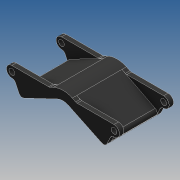
# Autodesk Inventor part: Front guard v2
Saved by Autodesk Inventor 2017 (Build 210142000, 142)
## iProperties
Created: 2017-07-08
Part Number: Front guard v2
Material: Generic
Document SubType Name: Modeling
Designer: yella
Density: 1 g/cm^3
Appearance: Rubber - Black
Author: yella
Autodesk Inventor part; units mm, degrees
ref_plane "YZ Plane" through (0, 0, 0) normal (1, 0, 0) x (0, 1, 0)
ref_plane "XZ Plane" through (0, 0, 0) normal (0, 1, 0) x (-1, 0, 0)
ref_plane "XY Plane" through (0, 0, 0) normal (0, 0, 1) x (1, 0, 0)
sketch "Sketch1" plane through (0, 0, 0) normal (0, 1, 0) x (-1, 0, 0)
  circle A0 centre (24, -57.282) radius 1.6
  circle A1 centre (-24, -57.282) radius 1.6
  circle A2 centre (30.6147, -73.9104) radius 1.6
  circle A3 centre (-30.6218, -73.9137) radius 1.6
  circle A4 centre (28.2679, -64.7457) radius 1.6
  circle A5 centre (-28.2698, -64.7417) radius 1.6
  line L0 (48.2265, -83.602) -> (45.2265, -83.602)
  line L1 (45.2265, -83.602) -> (45.2265, -77.602)
  line L2 (45.2265, -77.602) -> (48.2265, -77.602)
  line L3 (48.2265, -77.602) -> (48.2265, -83.602)
  line L4 (-45.2265, -83.602) -> (-48.2265, -83.602)
  line L5 (-48.2265, -83.602) -> (-48.2265, -77.602)
  line L6 (-48.2265, -77.602) -> (-45.2265, -77.602)
  line L7 (-45.2265, -77.602) -> (-45.2265, -83.602)
  line L8 (48.3297, -88.9468) -> (2.1402, -66.9602)
  line L9 (-2.1585, -66.9605) -> (-48.3297, -88.9468)
  arc A6 (2.1402, -66.9602) -> (-2.1585, -66.9605) centre (-0.0088, -71.4748) ccw
  line L10 (30.6147, -73.9104) -> (28.0518, -79.2944)
  line L11 (28.0518, -79.2944) -> (-28.0596, -79.2944)
  line L12 (-30.6218, -73.9137) -> (-28.0596, -79.2944)
  line L13 (-28.0596, -79.2944) -> (-28.9194, -77.4887)
  line L14 (28.0518, -79.2944) -> (28.9114, -77.4887)
  line L15 (2.9996, -65.1544) -> (21.6357, -74.0254)
  line L16 (-3.0185, -65.1549) -> (-21.6362, -74.0204)
  arc A7 (2.9996, -65.1544) -> (-3.0185, -65.1549) centre (-0.009, -71.4749) ccw
  line L17 (26.297, -68.8861) -> (23.4415, -74.885)
  line L18 (24.3011, -73.0791) -> (25.5905, -70.3703)
  line L19 (7.0641, -61.5516) -> (5.1491, -60.64)
  line L20 (-26.2983, -68.8819) -> (-24.3017, -73.0746)
  line L21 (-23.4419, -74.8803) -> (-25.5914, -70.3663)
  line L22 (-5.1677, -60.6408) -> (-7.0717, -61.5474)
  arc A8 (5.1491, -60.64) -> (-5.1677, -60.6408) centre (-0.0085, -71.4751) ccw
  arc A9 (28.2679, -67.7457) -> (28.2679, -61.7457) centre (28.2679, -64.7457) ccw
  line L23 (28.2679, -64.7457) -> (28.2679, -61.7457) construction
  line L24 (28.2679, -64.7457) -> (31.2679, -64.7457) construction
  line L25 (28.2679, -64.7457) -> (28.2679, -67.7457) construction
  line L26 (28.2679, -61.7457) -> (7.9237, -61.7457)
  line L27 (28.2679, -67.7457) -> (28.1029, -67.7457)
  arc A10 (-28.2698, -61.7417) -> (-28.2698, -67.7417) centre (-28.2698, -64.7417) ccw
  line L28 (-28.2698, -64.7417) -> (-28.2698, -61.7417) construction
  line L29 (-28.2698, -64.7417) -> (-25.2698, -64.7417) construction
  line L30 (-28.2698, -67.7417) -> (-28.104, -67.7417)
  line L31 (-28.2698, -61.7417) -> (-7.9316, -61.7417)
  arc A11 (21.6357, -74.0254) -> (24.3011, -73.0791) centre (22.4953, -72.2195) ccw
  arc A12 (-24.3017, -73.0746) -> (-21.6362, -74.0204) centre (-22.496, -72.2147) ccw
  arc A13 (-7.9316, -61.7417) -> (-7.0717, -61.5474) centre (-7.9316, -59.7417) ccw
  arc A14 (7.0641, -61.5516) -> (7.9237, -61.7457) centre (7.9237, -59.7457) ccw
  arc A15 (28.1029, -67.7457) -> (26.297, -68.8861) centre (28.1029, -69.7457) ccw
  arc A16 (-26.2983, -68.8819) -> (-28.104, -67.7417) centre (-28.104, -69.7417) ccw
  point P0 (0, 0)
  dimension "d0" = 3.2
  dimension "d1" = 6
  dimension "d2" = 6
  dimension "d3" = 5
  dimension "d4" = 2
  dimension "d5" = 7
  dimension "d6" = 5
  dimension "d7" = 12
  dimension "d8" = 3
  dimension "d9" = 90
  dimension "d10" = 180
  dimension "d11" = 3
  dimension "d12" = 90
  dimension "d13" = 2
  dimension "d14" = 2
  constraints: 64 end point, 22 point on circle, 18 tangent, 17 centre point, 16 point on line, 11 perpendicular, 6 parallel, 5 horizontal, 4 coincident, 4 equal radius
  measures "d0" diameter of A5
  measures "d1" distance of L1.start L2.start
  measures "d2" distance of L4.end L6.start
  measures "d3" radius of A6
  measures "d4" distance of L11.end L13.end
  measures "d5" radius of A7
  measures "d6" distance of L17.end L18.end
  measures "d7" radius of A8
  measures "d8" radius of A9
  measures "d9" angle of L24 L23
  measures "d10" angle of L23 L25
  measures "d11" radius of A10
  measures "d12" angle of L29 L28
  measures "d13" radius of A11
  measures "d14" radius of A15
extrude "Extrusion1" add sketch "Sketch1" along normal blind 2.5 contours A7 L16 A12 L20 A16 L30 A10 L31 A13 L22 A8 L19 A14 L26 A9 L27 A15 L17 A11 L15
sketch "Sketch2" plane through (0, 2.5, 0) normal (0, 1, 0) x (1, 0, 0)
  arc A0 (-5.1491, 60.64) -> (5.1677, 60.6408) centre (0.0085, 71.4751) ccw projected
  line L0 (-5.1491, 60.64) -> (-23.5723, 70.0963)
  line L1 (-24.3011, 73.0791) -> (-26.297, 68.8861) projected
  line L2 (5.1677, 60.6408) -> (23.5733, 70.0916)
  line L3 (26.2983, 68.8819) -> (24.3017, 73.0746) projected
  arc A1 (-21.6357, 74.0254) -> (-24.3011, 73.0791) centre (-22.4953, 72.2195) ccw projected
  line L4 (-24.4649, 72.7352) -> (-24.3011, 73.0791)
  arc A2 (-24.4649, 72.7352) -> (-23.5723, 70.0963) centre (-22.659, 71.8756) ccw
  line L5 (24.4655, 72.7306) -> (24.3017, 73.0746)
  arc A3 (23.5733, 70.0916) -> (24.4655, 72.7306) centre (22.6598, 71.8708) ccw
  arc A4 (24.3017, 73.0746) -> (21.6362, 74.0204) centre (22.496, 72.2147) ccw projected
  line L6 (21.6362, 74.0204) -> (3.0185, 65.1549) projected
  line L7 (-2.9996, 65.1544) -> (-21.6357, 74.0254) projected
  arc A5 (-2.9996, 65.1544) -> (3.0185, 65.1549) centre (0.009, 71.4749) ccw projected
  point P0 (0, 0)
  point P1 (-25.2991, 70.9826)
  point P2 (25.3, 70.9782)
  dimension "d17" = 2
  dimension "d18" = 2
  constraints: 8 end point, 5 tangent, 4 point on circle, 4 point on line, 2 centre point, 2 midpoint
  measures "d17" radius of A2
  measures "d18" radius of A3
extrude "Extrusion2" add sketch "Sketch2" along normal blind 25
sketch "Sketch3" plane through (0, 27.5, 0) normal (0, 1, 0) x (1, 0, 0)
  arc A0 (23.5733, 70.0916) -> (24.4655, 72.7306) centre (22.6598, 71.8708) ccw projected
  line L0 (23.5733, 70.0916) -> (5.1677, 60.6408) projected
  line L1 (5.1677, 60.6408) -> (7.0717, 61.5474) projected
  arc A1 (7.9316, 61.7417) -> (7.0717, 61.5474) centre (7.9316, 59.7417) ccw projected
  line L2 (7.9316, 61.7417) -> (28.2698, 61.7417) projected
  arc A2 (28.2698, 61.7417) -> (28.2698, 67.7417) centre (28.2698, 64.7417) ccw projected
  line L3 (28.2698, 67.7417) -> (28.104, 67.7417) projected
  arc A3 (26.2983, 68.8819) -> (28.104, 67.7417) centre (28.104, 69.7417) ccw projected
  line L4 (26.2983, 68.8819) -> (24.4655, 72.7306) projected
  circle A4 centre (28.2698, 64.7417) radius 1.6 projected
  arc A5 (-5.1491, 60.64) -> (5.1677, 60.6408) centre (0.0085, 71.4751) ccw projected
  line L5 (5.1677, 60.6408) -> (23.5733, 70.0916) projected
  arc A6 (23.5733, 70.0916) -> (24.4655, 72.7306) centre (22.6598, 71.8708) ccw projected
  line L6 (24.4655, 72.7306) -> (24.3017, 73.0746) projected
  arc A7 (24.3017, 73.0746) -> (21.6362, 74.0204) centre (22.496, 72.2147) ccw projected
  line L7 (21.6362, 74.0204) -> (3.0185, 65.1549) projected
  arc A8 (-2.9996, 65.1544) -> (3.0185, 65.1549) centre (0.009, 71.4749) ccw projected
  line L8 (-2.9996, 65.1544) -> (-21.6357, 74.0254) projected
  arc A9 (-21.6357, 74.0254) -> (-24.3011, 73.0791) centre (-22.4953, 72.2195) ccw projected
  line L9 (-24.3011, 73.0791) -> (-24.4649, 72.7352) projected
  arc A10 (-24.4649, 72.7352) -> (-23.5723, 70.0963) centre (-22.659, 71.8756) ccw projected
  line L10 (-23.5723, 70.0963) -> (-5.1491, 60.64) projected
  arc A11 (-24.4649, 72.7352) -> (-23.5723, 70.0963) centre (-22.659, 71.8756) ccw projected
  line L11 (-24.4649, 72.7352) -> (-26.297, 68.8861) projected
  arc A12 (-28.1029, 67.7457) -> (-26.297, 68.8861) centre (-28.1029, 69.7457) ccw projected
  line L12 (-28.1029, 67.7457) -> (-28.2679, 67.7457) projected
  arc A13 (-28.2679, 67.7457) -> (-28.2679, 61.7457) centre (-28.2679, 64.7457) ccw projected
  line L13 (-28.2679, 61.7457) -> (-7.9237, 61.7457) projected
  arc A14 (-7.0641, 61.5516) -> (-7.9237, 61.7457) centre (-7.9237, 59.7457) ccw projected
  line L14 (-7.0641, 61.5516) -> (-5.1491, 60.64) projected
  line L15 (-5.1491, 60.64) -> (-23.5723, 70.0963) projected
  circle A15 centre (-28.2679, 64.7457) radius 1.6 projected
  point P0 (0, 0)
extrude "Extrusion3" add sketch "Sketch3" along normal blind 2.5
body "Solid1"
